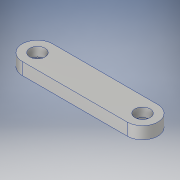
# Autodesk Inventor part: Linkage
Saved by Autodesk Inventor 2017 (Build 210142000, 142)
## iProperties
Created: 2017-02-08
Part Number: Linkage
Material: Aluminum 6061
Document SubType Name: Modeling
Designer: Joseph
Density: 2.7 g/cm^3
Appearance: Aluminum - Flat
Author: Joseph
Autodesk Inventor part; units mm, degrees
ref_plane "YZ Plane" through (0, 0, 0) normal (1, 0, 0) x (0, 1, 0)
ref_plane "XZ Plane" through (0, 0, 0) normal (0, 1, 0) x (-1, 0, 0)
ref_plane "XY Plane" through (0, 0, 0) normal (0, 0, 1) x (1, 0, 0)
sketch "Sketch1" plane through (0, 0, 0) normal (0, 1, 0) x (-1, 0, 0)
  line L0 (0, 0) -> (44.45, 0)
  line L1 (44.45, 0) -> (44.45, -10)
  line L2 (44.45, -10) -> (0, -10)
  line L3 (0, -10) -> (0, 0)
  dimension "d0" = 44.45
  dimension "d1" = 10
  constraints: 8 end point, 2 parallel, 1 horizontal, 1 perpendicular
  measures "d0" distance of L1.end L2.end
  measures "d1" distance of L0.end L1.end
extrude "Extrusion1" add sketch "Sketch1" along normal blind 4
sketch "Sketch2" plane through (0, 4, 0) normal (0, 1, 0) x (1, 0, 0)
  circle A0 centre (-39.45, 5) radius 2.5
  circle A1 centre (-5, 5) radius 2.5
  line L0 (-44.45, 10) -> (-44.45, 0) projected
  point P0 (0, 0)
  dimension "d4" = 5
  dimension "d5" = 5
  dimension "d6" = 5
  dimension "d7" = 5
  dimension "d8" = 5
  constraints: 2 centre point, 1 equal radius
  measures "d4" diameter of A0
  measures "d5" vertical distance of point (0, 0) A0.centre
  measures "d6" horizontal distance of point (0, 0) A1.centre
  measures "d7" horizontal distance of point (0, 0) A1.centre
  measures "d8" distance from line of L0 A0.centre
extrude "Extrusion2" cut sketch "Sketch2" against normal blind 3
fillet "Fillet1" radius 5 4 edges at (-44.45, 2, 0) (0, 2, 0) (0, 2, -10) (-44.45, 2, -10)
body "Solid1"
